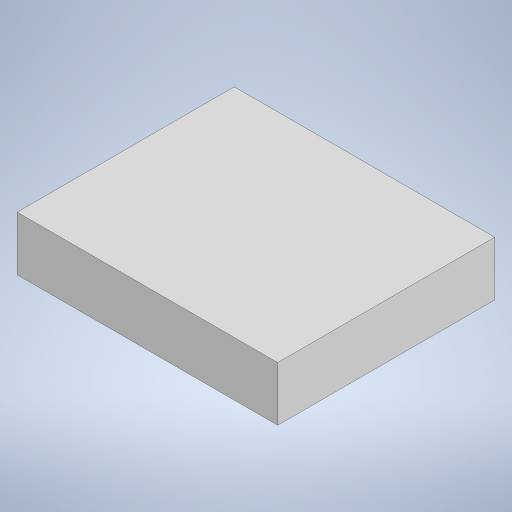
# Autodesk Inventor part: silicone glue
Saved by Autodesk Inventor 2024.2 (Build 282272000, 272)
## iProperties
Created: 2025-02-11
Part Number: silicone glue
Material: Generic
Document SubType Name: Modeling
Designer: Tom
Density: 1 g/cm^3
Appearance: Default
Author: Tom
Autodesk Inventor part; units mm, degrees
ref_plane "YZ Plane" through (0, 0, 0) normal (1, 0, 0) x (0, 1, 0)
ref_plane "XZ Plane" through (0, 0, 0) normal (0, 1, 0) x (-1, 0, 0)
ref_plane "XY Plane" through (0, 0, 0) normal (0, 0, 1) x (1, 0, 0)
sketch "Sketch1" plane through (0, 0, 0) normal (0, 1, 0) x (-1, 0, 0)
  line L0 (0, 0) -> (7.62, 0)
  line L1 (7.62, 0) -> (7.62, -6.35)
  line L2 (7.62, -6.35) -> (0, -6.35)
  line L3 (0, -6.35) -> (0, 0)
  dimension "d5" = 7.62
  dimension "d6" = 6.35
  constraints: 8 end point, 2 parallel, 1 horizontal, 1 perpendicular
  measures "d5" distance of L1.end L2.end
  measures "d6" distance of L2.end L0.start
extrude "Extrusion1" add sketch "Sketch1" along normal blind 1.5875
body "Solid1"
